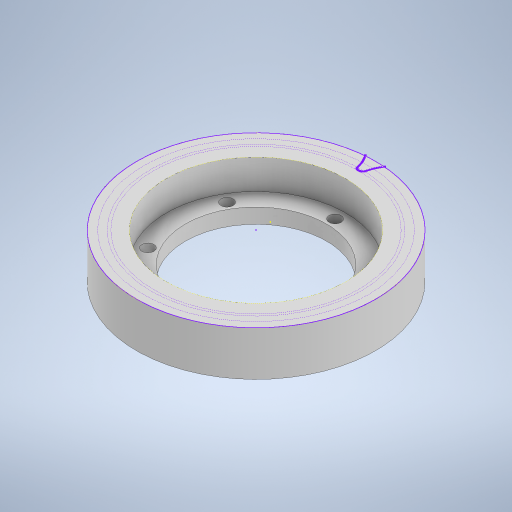
# Autodesk Inventor part: ZubkataiaBig
Saved by Autodesk Inventor 2024 (Build 280153000, 153)
## iProperties
Created: 2023-10-17
Part Number: ZubkataiaBig
Material: Generic
Document SubType Name: Modeling
Designer: Kippi
Density: 1 g/cm^3
Appearance: Default
Author: Kippi
Autodesk Inventor part; units mm, degrees
ref_plane "YZ Plane" through (0, 0, 0) normal (1, 0, 0) x (0, 1, 0)
ref_plane "XZ Plane" through (0, 0, 0) normal (0, 1, 0) x (-1, 0, 0)
ref_plane "XY Plane" through (0, 0, 0) normal (0, 0, 1) x (1, 0, 0)
sketch "Sketch1" plane through (0, 0, 0) normal (0, 1, 0) x (-1, 0, 0)
  circle A0 centre (0.0407, 9.5963) radius 62.5
  circle A1 centre (0.0407, 9.5963) radius 53
  circle A2 centre (0.0407, -43.4037) radius 4.05
  circle A3 centre (0.0407, 9.5963) radius 44
  circle A4 centre (45.9401, -16.9037) radius 4.05
  circle A5 centre (45.9401, 36.0963) radius 4.05
  circle A6 centre (0.0407, 62.5963) radius 4.05
  circle A7 centre (-45.8586, 36.0963) radius 4.05
  circle A8 centre (-45.8586, -16.9037) radius 4.05
  circle A9 centre (0.0407, 9.5963) radius 47.2699
  circle A10 centre (0.0407, 9.5963) radius 80.0292
  point P0 (0, 0)
  dimension "d3" = 106
  dimension "d2" = 125
  dimension "d4" = 360
  dimension "d5" = 8.1
  constraints: 10 centre point, 5 coincident, 1 vertical alignment, 15 other
  measures "d2" diameter of A0
  measures "d5" diameter of A2
extrude "Extrusion1" add sketch "Sketch1" along normal blind 30 contours A0 | A1 A4 A2 A8 A7 A6 A5 | A10
sketch "Sketch2" plane through (-0.0407, 30, 9.5963) normal (0, 1, 0) x (1, 0, 0)
  circle A0 centre (0, 0) radius 47.2699 construction
  circle A1 centre (0, 0) radius 60
  point P0 (0.0407, 9.5963)
  dimension "d8" = 120
  constraints: 1 centre point, 1 coincident
  measures "d8" diameter of A1
extrude "Extrusion2" cut sketch "Sketch2" against normal blind 20
sketch "Sketch4" plane through (-0.0407, 30, 9.5963) normal (0, 1, 0) x (1, 0, 0)
  circle A0 centre (0, 0) radius 60 construction
  circle A1 centre (0, 0) radius 80.0292 construction
  spline S0 degree 3 poles (-6.5259, 79.7334) (-6.2263, 79.2581) (-5.7769, 78.5452) (-5.2243, 77.5668) (-4.8273, 76.8235) (-4.451, 76.0694) (-4.0967, 75.3048) (-3.7666, 74.5294) (-3.4631, 73.7432) (-3.1905, 72.9457) (-2.9506, 72.1376) (-2.7945, 71.4528) (-2.6817, 70.9025) (-2.5626, 70.4977) (-2.4016, 70.1077) (-2.1917, 69.7409) (-1.9706, 69.4668) (-1.7708, 69.2687) (-1.6019, 69.1425) (-1.4288, 69.0215) (-1.2381, 68.9312) (-1.0444, 68.8474) (-0.8391, 68.7979) (-0.6323, 68.7561) (-0.3509, 68.7461) (0, 68.7526) (0.3509, 68.7461) (0.6323, 68.7561) (0.8391, 68.7979) (1.0444, 68.8474) (1.2381, 68.9312) (1.4288, 69.0215) (1.6019, 69.1425) (1.7708, 69.2687) (1.9706, 69.4668) (2.1917, 69.7409) (2.4016, 70.1077) (2.5626, 70.4977) (2.6817, 70.9025) (2.7945, 71.4528) (2.9506, 72.1376) (3.1905, 72.9457) (3.4631, 73.7432) (3.7666, 74.5294) (4.0967, 75.3048) (4.451, 76.0694) (4.8273, 76.8235) (5.2243, 77.5668) (5.7769, 78.5452) (6.2263, 79.2581) (6.5259, 79.7334) knots 0 0 0 0 0.168512 0.252773 0.337035 0.421295 0.505556 0.589816 0.674075 0.758333 0.842588 0.926838 0.968959 1.011074 1.053192 1.095291 1.137378 1.158442 1.179505 1.200561 1.221628 1.242684 1.263747 1.284807 1.305869 1.348 1.390132 1.411193 1.432253 1.453316 1.474372 1.495439 1.516495 1.537558 1.558622 1.60071 1.642808 1.684926 1.727041 1.769162 1.853412 1.937667 2.021925 2.106184 2.190444 2.274705 2.358966 2.443227 2.527488 2.696 2.696 2.696 2.696
  circle A2 centre (0, 0) radius 68.75 construction
  circle A3 centre (0, 0) radius 70.4769 construction
  circle A4 centre (0, 0) radius 75 construction
  circle A5 centre (0, 0) radius 80
  point P0 (0.0407, 9.5963)
  point P1 (-5.6426, 78.2983)
  point P2 (-5.2272, 77.5652)
  point P3 (-4.8307, 76.8217)
  point P4 (-4.4547, 76.0677)
  point P5 (-4.1007, 75.303)
  point P6 (-3.771, 74.5276)
  point P7 (-3.4682, 73.7413)
  point P8 (-3.1959, 72.9439)
  point P9 (-2.9594, 72.1353)
  point P10 (-2.7673, 71.315)
  point P11 (-2.676, 70.9038)
  point P12 (-2.5556, 70.5002)
  point P13 (-2.3934, 70.1115)
  point P14 (-2.1825, 69.7472)
  point P15 (-1.9188, 69.4191)
  point P16 (-1.7676, 69.2724)
  point P17 (-1.6012, 69.1434)
  point P18 (-1.4259, 69.0267)
  point P19 (-1.2376, 68.9322)
  point P20 (-1.0425, 68.8531)
  point P21 (-0.8389, 68.7992)
  point P22 (-0.6316, 68.7618)
  point P23 (-0.4213, 68.7499)
  point P24 (0, 68.75)
  point P25 (0.4213, 68.7499)
  point P26 (0.6316, 68.7618)
  point P27 (0.8389, 68.7992)
  point P28 (1.0425, 68.8531)
  point P29 (1.2376, 68.9322)
  point P30 (1.4259, 69.0267)
  point P31 (1.6012, 69.1434)
  point P32 (1.7676, 69.2724)
  point P33 (1.9188, 69.4191)
  point P34 (2.1825, 69.7472)
  point P35 (2.3934, 70.1115)
  point P36 (2.5556, 70.5002)
  point P37 (2.676, 70.9038)
  point P38 (2.7673, 71.315)
  point P39 (2.9594, 72.1353)
  point P40 (3.1959, 72.9439)
  point P41 (3.4682, 73.7413)
  point P42 (3.771, 74.5276)
  point P43 (4.1007, 75.303)
  point P44 (4.4547, 76.0677)
  point P45 (4.8307, 76.8217)
  point P46 (5.2272, 77.5652)
  point P47 (5.6426, 78.2983)
  constraints: 4 centre point, 2 point on circle, 49 other
body "Solid1"
